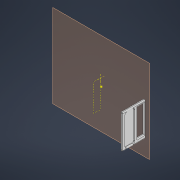
# Autodesk Inventor part: io_panel_adapter
Saved by Autodesk Inventor 2022 (Build 260153000, 153)
## iProperties
Created: 2025-02-02
Part Number: io_panel_adapter
Material: 一般
Document SubType Name: Modeling
Designer: nyxeon
Density: 1 g/cm^3
Appearance: 既定
Author: nyxeon
Autodesk Inventor part; units mm, degrees
ref_plane "YZ Plane" through (0, 0, 0) normal (1, 0, 0) x (0, 1, 0)
ref_plane "XZ Plane" through (0, 0, 0) normal (0, 1, 0) x (-1, 0, 0)
ref_plane "XY Plane" through (0, 0, 0) normal (0, 0, 1) x (1, 0, 0)
ref_plane "作業平面1" through (0, 0, 0) normal (0, 0, 1) x (1, 0, 0)
sketch "スケッチ4" plane through (0, 0, 0) normal (1, 0, 0) x (0, 1, 0)
  line L0 (-112.24, 47.221) -> (44.24, 47.221) construction
  line L1 (-113.34, 3.941) -> (-113.34, 46.121) construction
  line L2 (45.34, 46.121) -> (45.34, 3.941) construction
  line L3 (44.24, 2.841) -> (-112.24, 2.841) construction
  point P0 (0, 0)
  constraints: 1 other
sketch "スケッチ2" plane through (0, 0, 0) normal (0, 0, 1) x (1, 0, 0)
  circle A0 centre (250, -130) radius 2.1 construction
  circle A1 centre (250, 55) radius 2.1 construction
  circle A2 centre (250, -130) radius 2.25
  circle A3 centre (250, 55) radius 2.25
  line L0 (250, -130) -> (250, 55) construction
  line L1 (255, -130) -> (255, 55)
  line L2 (245, 55) -> (245, -130)
  arc A4 (245, -130) -> (255, -130) centre (250, -130) ccw
  arc A5 (255, 55) -> (245, 55) centre (250, 55) ccw
  point P0 (0, 0)
  point P1 (250, -37.5)
  dimension "d0" = 4.5
  dimension "d1" = 10
  constraints: 8 end point, 4 centre point, 4 point on circle, 4 tangent, 2 coincident, 1 equal radius, 1 midpoint, 1 parallel, 1 vertical
  measures "d0" diameter of A2
  measures "d1" diameter of A5
extrude "押し出し1" add sketch "スケッチ2" along normal blind 130
sketch "スケッチ3" plane through (255, -130, 0) normal (1, 0, 0) x (0, 0, -1)
  line L0 (-2.841, 175.34) -> (-47.221, 175.34)
  line L1 (-47.221, 175.34) -> (-47.221, 16.66)
  line L2 (-47.221, 16.66) -> (-2.841, 16.66)
  line L3 (-2.841, 16.66) -> (-2.841, 175.34)
  line L4 (-46.121, 175.34) -> (-3.941, 175.34) construction
  line L5 (-2.841, 174.24) -> (-2.841, 17.76) construction
  line L6 (-47.221, 17.76) -> (-47.221, 174.24) construction
  line L7 (-3.941, 16.66) -> (-46.121, 16.66) construction
  point P0 (0, 130)
  constraints: 8 end point, 4 point on line, 2 parallel, 1 horizontal, 1 perpendicular
extrude "押し出し2" cut sketch "スケッチ3" along normal through all both and the other way through all
sketch "スケッチ5" plane through (0, 0, 130) normal (0, 0, 1) x (1, 0, 0)
  arc A0 (255, 55) -> (245, 55) centre (250, 55) ccw projected
  line L0 (245, 55) -> (245, -130) projected
  arc A1 (245, -130) -> (255, -130) centre (250, -130) ccw projected
  line L1 (245, -130) -> (245, -135)
  line L2 (245, -135) -> (250, -135)
  line L3 (245, 55) -> (245, 60)
  line L4 (245, 60) -> (250, 60)
  arc A2 (255, 55) -> (245, 55) centre (250, 55) ccw projected
  point P0 (0, 0)
  constraints: 8 end point, 3 point on circle, 2 horizontal, 2 vertical
extrude "押し出し3" add sketch "スケッチ5" against normal up to surface (130 mm away)
sketch "スケッチ6" plane through (255, -130, 0) normal (1, 0, 0) x (0, 0, -1)
  line L0 (-59.221, 180) -> (-118, 180)
  line L1 (-118, 180) -> (-118, 5)
  line L2 (-118, 5) -> (-59.221, 5)
  line L3 (-59.221, 5) -> (-59.221, 180)
  line L4 (0, 185) -> (-130, 185) projected
  line L5 (0, 0) -> (-130, 0) projected
  line L6 (-130, 0) -> (-130, 185) projected
  line L7 (-47.221, 16.66) -> (-47.221, 175.34) projected
  point P0 (0, 130)
  dimension "d8" = 5
  dimension "d9" = 5
  dimension "d10" = 12
  dimension "d11" = 12
  constraints: 8 end point, 2 parallel, 1 horizontal, 1 perpendicular
  measures "d8" distance between parallel lines of L0 L4
  measures "d9" distance between parallel lines of L5 L2
  measures "d10" distance between parallel lines of L6 L1
  measures "d11" distance between parallel lines of L7 L3
extrude "押し出し4" cut sketch "スケッチ6" against normal blind 8
fillet "フィレット1" radius 5 2 edges at (255, 50, 88.6105) (255, -125, 88.6105)
fillet "フィレット2" radius 10 8 edges at (248.5001, 50, 59.221) (248.5001, 50, 118) (253.5356, 51.4644, 118) (253.5356, 51.4644, 59.221) (253.5356, -126.4644, 59.221) (248.5001, -125, 59.221) (248.5001, -125, 118) (253.5356, -126.4644, 118)
sketch "スケッチ7" plane through (0, 0, 130) normal (0, 0, 1) x (1, 0, 0)
  line L0 (245, 60) -> (245, -135) projected
  line L1 (245.3, 60) -> (245.3, -135)
  line L2 (245.3, -135) -> (245, -135)
  line L3 (245.3, 60) -> (245, 60)
  point P0 (0, 0)
  dimension "d16" = 0.3
  constraints: 6 end point, 2 horizontal, 1 parallel
  measures "d16" distance between parallel lines of L0 L1
extrude "押し出し5" cut sketch "スケッチ7" against normal through all
fillet "フィレット3" radius 5 2 edges at (255, -113.34, 25.031) (255, 45.34, 25.031)
equation "\"d9\" = d8"
equation "\"d11\" = d10"
